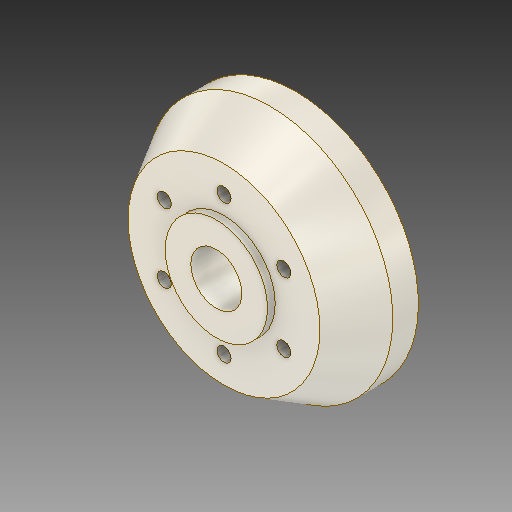
# Autodesk Inventor part: 301-08
Saved by Autodesk Inventor 2019 (Build 230136000, 136)
## iProperties
Company: Autodesk Inc.
Created: 2017-06-23
Part Number: 301-08
Material: Titanium
Document SubType Name: Modeling
Designer: Autodesk Inc.
Density: 4.51 g/cm^3
Appearance: Titanium
Mass: 417.03 g
Surface Area: 288.786 cm^2
Volume: 92.4678 cm^3
Author: Inventor
Autodesk Inventor part; units mm, degrees
ref_plane "YZ Plane" through (0, 0, 0) normal (1, 0, 0) x (0, 1, 0)
ref_plane "XZ Plane" through (0, 0, 0) normal (0, 1, 0) x (-1, 0, 0)
ref_plane "XY Plane" through (0, 0, 0) normal (0, 0, 1) x (1, 0, 0)
sketch "Sketch1" plane through (0, 0, 0) normal (1, 0, 0) x (0, 1, 0)
  line L0 (0, 0) -> (0, -18)
  line L1 (37.5, 0) -> (48, -18)
  line L2 (37.5, 0) -> (0, 0)
  line L3 (46, -18.5407) -> (41.0179, -10)
  line L4 (41.0179, -10) -> (37.5, -10)
  line L5 (46, -18.5407) -> (46, -28)
  line L6 (46, -28) -> (48, -28)
  line L7 (48, -28) -> (48, -18)
  line L8 (0, -18) -> (37.5, -18)
  line L9 (37.5, -18) -> (37.5, -10)
  dimension "d0" = 18
  dimension "d6" = 75
  dimension "d7" = 96
  dimension "d9" = 10
  dimension "d10" = 10
  dimension "d11" = 2
  dimension "d12" = 2
  constraints: 20 end point, 4 horizontal, 3 vertical, 2 horizontal alignment, 2 parallel, 1 vertical alignment
  measures "d0" distance of L0.start L0.end
  measures "d6" diameter of L1.start L0
  measures "d7" diameter of L1.end L0
  measures "d9" distance between parallel lines of L2 L4
  measures "d10" distance of L6.end L1.end
  measures "d11" distance of L5.end L6.end
  measures "d12" distance between parallel lines of L1 L3
revolve "Revolution1" add sketch "Sketch1" angle 360 about axis through (0, 0, 0) along (0, 0, -1)
sketch "Sketch2" plane through (0, 0, 0) normal (0, 0, 1) x (1, 0, 0)
  circle A0 centre (0, 0) radius 20
  point P0 (0, 0)
  dimension "d14" = 40
  constraints: 1 centre point, 1 coincident
  measures "d14" diameter of A0
extrude "Extrusion1" add sketch "Sketch2" along normal blind 3
sketch "Sketch3" plane through (0, 0, -18) normal (0, 0, -1) x (-1, 0, 0)
  circle A0 centre (0, 0) radius 10
  point P0 (0, 0)
  dimension "d17" = 20
  constraints: 1 centre point, 1 coincident
  measures "d17" diameter of A0
extrude "Extrusion2" cut sketch "Sketch3" against normal through all
sketch "Sketch4" plane through (0, 0, 0) normal (0, 0, 1) x (1, 0, 0)
  circle A0 centre (0, 27) radius 2.065
  point P0 (0, 0)
  dimension "d20" = 27
  constraints: 1 centre point
  measures "d20" distance of A0.centre point (0, 0)
hole "Hole1" at (0, 27, 0) direction (0, 0, -1) diameter 5.5 end through all
thread "Thread2" size "M5.5x0.5" class "6H" standard "ANSI Metric M Profile" full length
pattern_circular "Circular Pattern1" count 6 over 360 about axis through (0, 0, -9) along (0, 0, -1) of "Hole1"
body "Solid1"
